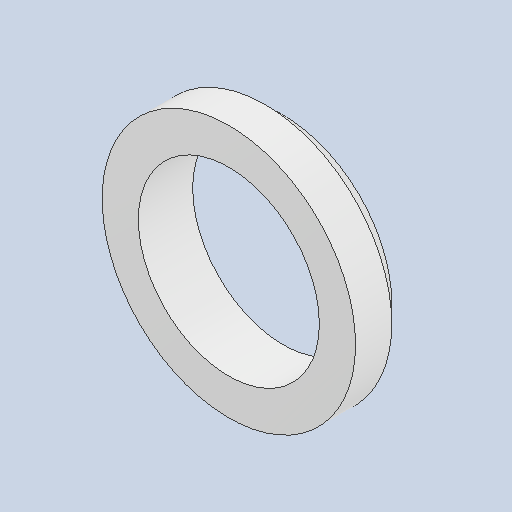
# Autodesk Inventor part: w1.5f5-7n
Saved by Autodesk Inventor 2023 (Build 270158030, 158C)
## iProperties
Created: 2022-01-09
Part Number: w1.5f5-7n
Material: アセタール樹脂、白
Document SubType Name: Modeling
Designer: acps
Density: 1.425 g/cm^3
Appearance: 滑らか - 白
Mass: 0.0365603 g
Surface Area: 0.874814 cm^2
Volume: 0.0256563 cm^3
Author: acps
Autodesk Inventor part; units mm, degrees
ref_plane "YZ Plane" through (0, 0, 0) normal (1, 0, 0) x (0, 1, 0)
ref_plane "XZ Plane" through (0, 0, 0) normal (0, 1, 0) x (-1, 0, 0)
ref_plane "XY Plane" through (0, 0, 0) normal (0, 0, 1) x (1, 0, 0)
sketch "Sketch1" plane through (0, 0, 0) normal (0, 0, 1) x (1, 0, 0)
  circle A0 centre (0, 0) radius 2.5
  circle A1 centre (0, 0) radius 3.5
  dimension "d0" = 5
  dimension "d1" = 7
  constraints: 2 centre point, 2 coincident
  measures "d0" diameter of A0
  measures "d1" diameter of A1
extrude "Extrusion1" add sketch "Sketch1" against normal blind 1.5
chamfer "Chamfer1" distance 0.5 angle 45 1 edges at (-3.5, 0, -1.5)
body "Solid1"
